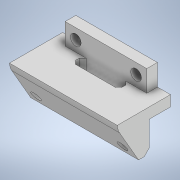
# Autodesk Inventor part: ultrasonic mount to deadbolt enclosure
Saved by Autodesk Inventor 2022 (Build 260153000, 153)
## iProperties
Created: 2022-04-07
Part Number: ultrasonic mount to deadbolt enclosure
Material: Generic
Document SubType Name: Modeling
Designer: a-dubs
Density: 1 g/cm^3
Appearance: Default
Author: a-dubs
Autodesk Inventor part; units mm, degrees
ref_plane "YZ Plane" through (0, 0, 0) normal (1, 0, 0) x (0, 1, 0)
ref_plane "XZ Plane" through (0, 0, 0) normal (0, 1, 0) x (-1, 0, 0)
ref_plane "XY Plane" through (0, 0, 0) normal (0, 0, 1) x (1, 0, 0)
sketch "Sketch2" plane through (0, 0, 0) normal (0, 0, 1) x (1, 0, 0)
  line L0 (0, 0) -> (18.13, 0)
  circle A0 centre (0, 0) radius 1.6
  circle A1 centre (18.13, 0) radius 1.6
  line L1 (0, 0) -> (-3.2, 0)
  line L2 (-3.2, 0) -> (-3.2, -3.2)
  line L3 (9.065, 0) -> (9.065, -3.2)
  line L4 (-3.2, 0) -> (-3.2, 3.2)
  line L5 (-3.2, 3.2) -> (9.065, 3.2)
  line L6 (9.065, 3.2) -> (18.13, 3.2)
  line L7 (18.13, 3.2) -> (21.33, 3.2)
  line L8 (21.33, 3.2) -> (21.33, -3.2)
  line L9 (9.065, -3.2) -> (22.065, -3.2)
  line L10 (22.065, -3.2) -> (25.265, -3.2)
  line L11 (25.265, -3.2) -> (25.265, -6.4)
  line L12 (25.265, -6.4) -> (9.065, -6.4)
  line L13 (9.065, -3.2) -> (9.065, -6.4)
  line L14 (9.065, -3.2) -> (-3.935, -3.2)
  line L15 (-3.935, -3.2) -> (-7.135, -3.2)
  line L16 (-7.135, -3.2) -> (-7.135, -6.4)
  line L17 (-7.135, -6.4) -> (9.065, -6.4)
  dimension "d10" = 18.13
  dimension "d11" = 3.2
  dimension "d12" = 3.2
  dimension "d13" = 3.2
  dimension "d16" = 3.2
  dimension "d19" = 13
  constraints: 36 end point, 4 horizontal, 4 perpendicular, 4 point on line, 3 symmetric about line, 2 centre point, 2 coincident, 2 vertical, 1 midpoint
  measures "d10" distance of L0.start L0.end
  measures "d11" diameter of A0
  measures "d12" diameter of A1
  measures "d13" distance of L1.start L1.end
  measures "d16" distance of L6.end L7.end
  measures "d19" distance of L3.end L9.end
extrude "Extrusion1" add sketch "Sketch2" along normal blind 3.2 contours A0 L1 L4 L5 L6 L7 L8 L9 L3 L0 | L0 L3 L14 L2 L1 A0
extrude "Extrusion2" add sketch "Sketch2" along normal blind 16 contours L9 L10 L11 L12 L13 | L13 L17 L16 L15 L14
sketch "Sketch3" plane through (-7.135, -6.4, 0) normal (0, -1, 0) x (1, 0, 0)
  line L0 (0, 0) -> (0, 16) projected
  line L1 (32.4, 0) -> (32.4, 16) projected
  line L2 (0, 16) -> (32.4, 16)
  line L3 (32.4, 16) -> (32.4, 9.6)
  line L4 (32.4, 9.6) -> (0, 9.6)
  line L5 (0, 0) -> (0, 16) projected
  line L6 (32.4, 16) -> (0, 16) projected
  line L7 (0, 16) -> (0, 9.6)
  line L8 (16.2, 9.6) -> (16.2, 16)
  point P0 (7.135, 0)
  point P1 (0, 9.6)
  dimension "d26" = 6.4
  constraints: 10 end point, 2 midpoint, 2 point on line, 1 collinear, 1 horizontal, 1 perpendicular
  measures "d26" distance of L1.end L3.end
extrude "Extrusion3" add sketch "Sketch3" along normal blind 9
draft "FaceDraft1" angle 60 pull direction (0, 0, 1) faces at (3.665, -15.4, 13.8667) fixed edges at (9.065, -15.4, 9.6)
sketch "Sketch4" plane through (-7.135, -4.3149, 16) normal (0, -0.5, 0.8660254) x (1, 0, 0)
  line L0 (0, -5.0058) -> (0, -12.8) projected
  line L1 (0, -12.8) -> (32.4, -12.8) projected
  line L2 (0, -12.8) -> (32.4, -12.8)
  line L3 (16.2, -12.8) -> (3.2, -12.8)
  line L4 (3.2, -12.8) -> (3.2, -9.6)
  circle A0 centre (3.2, -9.6) radius 1.45
  line L5 (16.2, -12.8) -> (16.2, -9.6)
  line L6 (29.2, -12.8) -> (29.2, -9.6)
  circle A1 centre (29.2, -9.6) radius 1.45
  point P0 (7.135, -4.2632)
  dimension "d30" = 13
  dimension "d31" = 3.2
  dimension "d32" = 2.9
  constraints: 10 end point, 3 symmetric about line, 2 centre point, 2 coincident, 1 collinear, 1 midpoint, 1 perpendicular, 1 point on line, 1 vertical, 1 other
  measures "d30" distance of L3.start L3.end
  measures "d31" distance of L3.end L4.end
  measures "d32" diameter of A0
sketch "Sketch5" plane through (25.265, -6.4, 9.6) normal (0, 0, -1) x (-1, 0, 0)
  line L0 (32.4, 2.0851) -> (32.4, -9) projected
  line L1 (0, 3.8) -> (32.4, 3.8)
  line L2 (32.4, 3.8) -> (32.4, -9)
  line L3 (32.4, -9) -> (0, -9)
  line L4 (0, -9) -> (0, 3.8)
  line L5 (0, 0) -> (0, -9) projected
  line L6 (0, 0) -> (32.4, 0)
  point P0 (25.265, 6.4)
  point P1 (32.4, 2.0851)
  constraints: 10 end point, 2 parallel, 1 horizontal, 1 perpendicular
extrude "Extrusion4" add sketch "Sketch5" along normal blind 3.2 contours L0 L3 L4 L6
extrude "Extrusion5" cut sketch "Sketch4" against normal up to surface surface through (9.065, -10.9, 6.4) normal (0, 0, -1)
fillet "Fillet1" radius 5 1 edges at (9.065, -4.3149, 16)
chamfer "Chamfer1" distance 1.5 angle 45 1 edges at (9.065, -15.4, 6.4)
sketch "Sketch6" plane through (-7.135, -6.4, 0) normal (0, -1, 0) x (1, 0, 0)
  line L0 (0, 0) -> (32.4, 0) projected
  line L1 (0, 0) -> (32.4, 0)
  line L2 (32.4, 0) -> (16.2, 0)
  line L3 (16.2, 0) -> (16.2, 6.4)
  line L4 (0, 6.4) -> (32.4, 6.4) projected
  line L5 (3.935, 3.2) -> (28.465, 3.2) projected
  line L6 (16.2, 3.2) -> (23.2, 3.2)
  line L7 (16.2, 3.2) -> (9.2, 3.2)
  line L8 (9.2, 3.2) -> (9.2, 6.4)
  line L9 (23.2, 3.2) -> (23.2, 6.4)
  line L10 (23.2, 6.4) -> (9.2, 6.4)
  point P0 (7.135, 0)
  dimension "d41" = 7
  dimension "d42" = 7
  constraints: 16 end point, 4 point on line, 3 midpoint, 2 collinear, 2 perpendicular
  measures "d41" distance of L6.start L6.end
  measures "d42" distance of L6.start L7.end
extrude "Extrusion6" cut sketch "Sketch6" against normal through all
chamfer "Chamfer2" distance 1 angle 45 4 edges at (2.065, -4.8, 6.4) (2.065, -4.8, 3.2) (16.065, -4.8, 6.4) (16.065, -4.8, 3.2)
body "Solid1"
